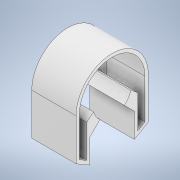
# Autodesk Inventor part: Brazo 3D
Saved by Autodesk Inventor 2022.2 (Build 262287010, 287A)
## iProperties
Created: 2022-10-08
Part Number: Brazo 3D
Material: Generic
Document SubType Name: Modeling
Designer: User
Density: 1 g/cm^3
Appearance: Flat - Gray 1
Author: User
Autodesk Inventor part; units mm, degrees
ref_plane "YZ Plane" through (0, 0, 0) normal (1, 0, 0) x (0, 1, 0)
ref_plane "XZ Plane" through (0, 0, 0) normal (0, 1, 0) x (-1, 0, 0)
ref_plane "XY Plane" through (0, 0, 0) normal (0, 0, 1) x (1, 0, 0)
sketch "Sketch1" plane through (0, 0, 0) normal (1, 0, 0) x (0, 1, 0)
  arc A0 (0, -65) -> (0, 65) centre (0, 0) ccw
  line L0 (0, 65) -> (-75, 65)
  line L1 (0, -65) -> (-75, -65)
  line L2 (-75, 65) -> (-95.2073, 30)
  line L3 (-75, 65) -> (-34.5855, 65) construction
  circle A1 centre (0, 0) radius 35
  line L4 (-95.2073, 40) -> (-45.2073, 40)
  line L5 (-45.2073, 40) -> (-27.215, 22.0078)
  line L6 (-45.2073, 40) -> (-19.7624, 40) construction
  line L7 (91.7333, 0) -> (-104.2658, 0) construction
  line L8 (-95.2073, -40) -> (-45.2073, -40)
  line L9 (-45.2073, -40) -> (-27.215, -22.0078)
  line L10 (-45.2073, -40) -> (-19.7624, -40) construction
  line L11 (-75, -65) -> (-95.2073, -30)
  circle A2 centre (0, 0) radius 29
  line L12 (-71.5359, 59) -> (0, 59)
  arc A3 (0, -59) -> (0, 59) centre (0, 0) ccw
  line L13 (0, -59) -> (-71.5359, -59)
  line L14 (-71.5359, 59) -> (-79.0415, 46)
  line L15 (-79.0415, 46) -> (-19.3504, 46)
  line L16 (-19.3504, 46) -> (-9.4012, 33.7138)
  line L17 (-71.5359, -59) -> (-79.0415, -46)
  line L18 (-79.0415, -46) -> (-19.3504, -46)
  line L19 (-19.3504, -46) -> (-9.4012, -33.7138)
  point P0 (-27.215, -22.0078)
  point P1 (-89.4338, -40)
  point P2 (-89.4338, 40)
  point P3 (-9.4012, -33.7138)
  dimension "d0" = 130
  dimension "d2" = 75
  dimension "d3" = 120
  dimension "d4" = 35
  dimension "d9" = 30
  dimension "d10" = 50
  dimension "d11" = 45
  dimension "d12" = 60
  dimension "d13" = 40
  dimension "d14" = 3.6821
  dimension "d15" = 68.5473
  dimension "d16" = 70.045
  dimension "d17" = 6
  dimension "d18" = 6
  dimension "d19" = 6
  dimension "d20" = 6
  dimension "d21" = 6
  dimension "d22" = 15.8094
  constraints: 40 end point, 8 symmetric about line, 7 horizontal, 6 point on circle, 4 centre point, 3 coincident, 3 equal length, 2 tangent, 2 other
  measures "d0" diameter of A0
  measures "d2" distance of L0.start L0.end
  measures "d3" angle of L2 L3
  measures "d4" vertical distance of L0.end L2.end
  measures "d9" radial gap between concentric circles of A0 A1
  measures "d10" distance of L4.start L4.end
  measures "d11" angle of L5 L6
  measures "d12" angle of L7 L11
  measures "d13" distance between parallel lines of L7 L6
  measures "d14" distance from line of point (0, 0) L5
  measures "d15" distance from line of L7.start L5
  measures "d16" distance from line of L7.end L5
  measures "d17" radial gap between concentric circles of A1 A2
  measures "d18" radial gap between concentric circles of A0 A3
  measures "d19" distance between parallel lines of L14 L2
  measures "d20" distance between parallel lines of L15 L4
  measures "d21" angle of L16 L5
  measures "d22" distance of L15.end L16.end
extrude "Extrusion3" add sketch "Sketch1" along normal blind 80 contours L1 L11 L8 L9 A1 L19 L18 L17 L13 A3 L12 L14 L15 L16 L5 L4 L2 L0 A0
extrude "Extrusion4" add sketch "Sketch1" along normal blind 10 contours A1 | A1 L16 L15 L14 L12 A3 L13 L17 L18 L19
body "Solid2"
